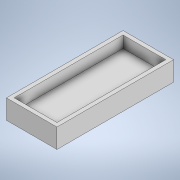
# Autodesk Inventor part: reed-switch-compartment
Saved by Autodesk Inventor 2021 (Build 250183000, 183)
## iProperties
Created: 2021-01-17
Part Number: reed-switch-compartment
Material: Generic
Document SubType Name: Modeling
Designer: Luke Kamols
Density: 1 g/cm^3
Appearance: Default
Author: Luke Kamols
Autodesk Inventor part; units mm, degrees
ref_plane "YZ Plane" through (0, 0, 0) normal (1, 0, 0) x (0, 1, 0)
ref_plane "XZ Plane" through (0, 0, 0) normal (0, 1, 0) x (-1, 0, 0)
ref_plane "XY Plane" through (0, 0, 0) normal (0, 0, 1) x (1, 0, 0)
sketch "Sketch1" plane through (0, 0, 0) normal (0, 1, 0) x (-1, 0, 0)
  line L0 (0, 0) -> (0, -30)
  line L1 (0, -30) -> (13, -30)
  line L2 (13, -30) -> (13, 0)
  line L3 (13, 0) -> (0, 0)
  dimension "d0" = 30
  dimension "d1" = 13
  constraints: 8 end point, 3 perpendicular, 1 vertical
  measures "d0" distance of L0.start L0.end
  measures "d1" distance of L0.end L1.end
extrude "Extrusion1" add sketch "Sketch1" along normal blind 2
sketch "Sketch2" plane through (0, 2, 0) normal (0, 1, 0) x (1, 0, 0)
  line L0 (-13, 30) -> (-13, 0) projected
  line L1 (0, 30) -> (-13, 30) projected
  line L2 (-13, 30) -> (-13, 0) projected
  line L3 (-13, 0) -> (0, 0) projected
  line L4 (0, 0) -> (0, 30) projected
  line L5 (0, 0) -> (0, 30) projected
  line L6 (0, 0) -> (0, 3)
  line L7 (-13, 30) -> (-13, 29)
  line L8 (-13, 29) -> (-12, 29)
  line L9 (-12, 29) -> (-1, 29)
  line L10 (-1, 29) -> (-1, 1)
  line L11 (-1, 1) -> (-12, 1)
  line L12 (-12, 1) -> (-12, 29)
  dimension "d13" = 1
  dimension "d14" = 1
  dimension "d15" = 11
  dimension "d16" = 28
  constraints: 14 end point, 2 parallel, 2 perpendicular, 2 point on line, 1 horizontal
  measures "d13" distance of L1.end L7.end
  measures "d14" distance of L7.end L8.end
  measures "d15" distance of L10.end L11.end
  measures "d16" distance of L9.end L10.end
extrude "Extrusion2" add sketch "Sketch2" along normal blind 3
body "Solid1"
